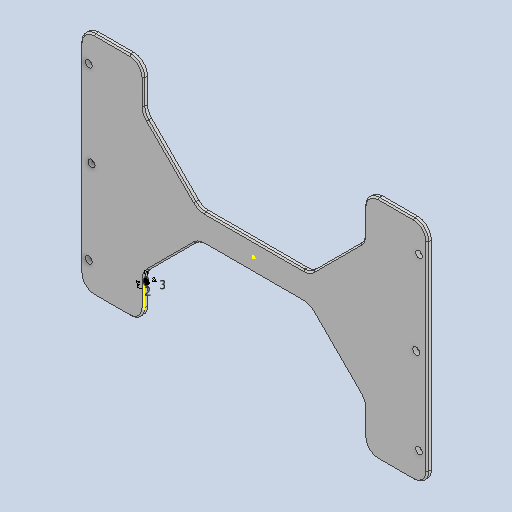
# Autodesk Inventor part: Holder
Saved by Autodesk Inventor 2022 (Build 260153000, 153)
## iProperties
Created: 2021-04-26
Part Number: Holder
Material: Generic
Document SubType Name: Modeling
Designer: lgnds
Density: 1 g/cm^3
Appearance: Default
Author: lgnds
Autodesk Inventor part; units mm, degrees
ref_plane "YZ Plane" through (0, 0, 0) normal (1, 0, 0) x (0, 1, 0)
ref_plane "XZ Plane" through (0, 0, 0) normal (0, 1, 0) x (-1, 0, 0)
ref_plane "XY Plane" through (0, 0, 0) normal (0, 0, 1) x (1, 0, 0)
sketch "Sketch1" plane through (0, 0, 0) normal (0, 0, 1) x (1, 0, 0)
  line L0 (-125.5, -82) -> (125.5, -82)
  line L1 (125.5, -82) -> (125.5, 82)
  line L2 (125.5, 82) -> (-125.5, 82)
  line L3 (-125.5, 82) -> (-125.5, -82)
  line L4 (-125.5, -82) -> (125.5, 82) construction
  line L5 (125.5, -82) -> (-125.5, 82) construction
  point P0 (0, 0)
  dimension "d0" = 251
  dimension "d1" = 164
  constraints: 12 end point, 2 midpoint, 2 parallel, 1 horizontal, 1 perpendicular
  measures "d0" distance of L1.end L2.end
  measures "d1" distance of L2.end L0.start
extrude "Extrusion1" add sketch "Sketch1" along normal blind 3
sketch "Sketch2" plane through (0, 0, 3) normal (0, 0, 1) x (1, 0, 0)
  line L0 (-245.98, 0) -> (245.98, 0) construction
  circle A0 centre (-117.5, 0) radius 2.6
  line L1 (-125.5, 82) -> (-125.5, -82) projected
  line L2 (0, -114.8) -> (0, 114.8) construction
  line L3 (245.98, 0) -> (-245.98, 0) construction
  circle A1 centre (117.5, 0) radius 2.6
  line L4 (-80, 82) -> (0, 82)
  line L5 (0, 82) -> (0, 10)
  line L6 (0, 10) -> (-80, 10)
  line L7 (-80, 10) -> (-80, 82)
  line L8 (80, 82) -> (0, 82)
  line L9 (0, 10) -> (80, 10)
  line L10 (80, 10) -> (80, 82)
  line L11 (-80, -82) -> (0, -82)
  line L12 (0, -82) -> (0, -10)
  line L13 (0, -10) -> (-80, -10)
  line L14 (-80, -10) -> (-80, -82)
  line L15 (80, -82) -> (0, -82)
  line L16 (0, -10) -> (80, -10)
  line L17 (80, -10) -> (80, -82)
  line L18 (125.5, 82) -> (-125.5, 82) projected
  point P0 (0, 0)
  dimension "d4" = 5.2
  dimension "d5" = 8
  dimension "d6" = 160
  dimension "d7" = 20
  constraints: 30 end point, 11 symmetric about line, 4 point on line, 2 centre point, 2 parallel, 1 horizontal, 1 perpendicular, 1 other
  measures "d4" diameter of A0
  measures "d5" distance from line of L1 A0.centre
  measures "d6" distance between parallel lines of L10 L7
  measures "d7" distance between parallel lines of L16 L9
extrude "Extrusion2" cut sketch "Sketch2" against normal through all
chamfer "Chamfer1" distance 40 angle 45 4 edges at (-80, 10, 1.5) (80, 10, 1.5) (80, -10, 1.5) (-80, -10, 1.5)
fillet "Fillet1" radius 10 16 edges at (-80, -50, 1.5) (-40, -10, 1.5) (-80, -82, 1.5) (-125.5, -82, 1.5) (-125.5, 82, 1.5) (-80, 82, 1.5) (-80, 50, 1.5) (-40, 10, 1.5) (40, 10, 1.5) (80, 50, 1.5) (80, 82, 1.5) (125.5, 82, 1.5) (125.5, -82, 1.5) (80, -82, 1.5) (80, -50, 1.5) (40, -10, 1.5)
chamfer "Chamfer2" distance 1 angle 45 32 edges at (-82.9289, -79.0711, 3) (-102.75, -82, 3) (-122.5711, -79.0711, 3) (-125.5, 0, 3) (-122.5711, 79.0711, 3) (-102.75, 82, 3) (-82.9289, 79.0711, 3) (-80, 63.0711, 3) (-79.2388, 50.3153, 3) (-60, 30, 3) (-39.6847, 10.7612, 3) (0, 10, 3) (39.6847, 10.7612, 3) (60, 30, 3) (79.2388, 50.3153, 3) (80, 63.0711, 3) (82.9289, 79.0711, 3) (102.75, 82, 3) (122.5711, 79.0711, 3) (125.5, 0, 3) (122.5711, -79.0711, 3) (102.75, -82, 3) (82.9289, -79.0711, 3) (80, -63.0711, 3) (79.2388, -50.3153, 3) (60, -30, 3) (39.6847, -10.7612, 3) (0, -10, 3) (-39.6847, -10.7612, 3) (-60, -30, 3) (-79.2388, -50.3153, 3) (-80, -63.0711, 3)
sketch "Sketch3" plane through (0, 0, 3) normal (0, 0, 1) x (1, 0, 0)
  circle A0 centre (-119.5, 61.5) radius 2.5
  line L0 (-175.7, 0) -> (175.7, 0) projected
  line L1 (0, -114.8) -> (0, 114.8) construction
  circle A1 centre (119.5, 61.5) radius 2.5
  circle A2 centre (-119.5, -61.5) radius 2.5
  circle A3 centre (119.5, -61.5) radius 2.5
  point P0 (0, 0)
  dimension "d17" = 5
  dimension "d18" = 123
  dimension "d19" = 239
  constraints: 4 centre point, 3 symmetric about line, 3 other
  measures "d17" diameter of A0
  measures "d18" distance of A2.centre A0.centre
  measures "d19" distance of A1.centre A0.centre
extrude "Extrusion3" cut sketch "Sketch3" against normal through all
sketch "Sketch4" plane through (0, 0, 3) normal (0, 0, 1) x (1, 0, 0)
  circle A0 centre (-78, -54.1421) radius 1.5
  line L0 (-80, -72) -> (-80, -54.1421) projected
  point P0 (0, 0)
  dimension "d22" = 3
  dimension "d23" = 2
  dimension "d24" = 0
  constraints: 1 centre point
  measures "d22" diameter of A0
  measures "d23" distance from line of L0 A0.centre
  measures "d24" vertical distance of L0.end A0.centre
body "Solid1"
